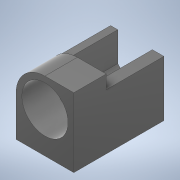
# Autodesk Inventor part: MotorMountV1
Saved by Autodesk Inventor 2020 (Build 240168000, 168)
## iProperties
Created: 2023-11-27
Part Number: MotorMountV1
Material: Thermoplastic Resin
Document SubType Name: Modeling
Designer: smz3rm
Density: 1.28 g/cm^3
Appearance: Smooth - Black
Author: smz3rm
Autodesk Inventor part; units mm, degrees
ref_plane "YZ Plane" through (0, 0, 0) normal (1, 0, 0) x (0, 1, 0)
ref_plane "XZ Plane" through (0, 0, 0) normal (0, 1, 0) x (-1, 0, 0)
ref_plane "XY Plane" through (0, 0, 0) normal (0, 0, 1) x (1, 0, 0)
sketch "Sketch4" plane through (0, 0, 0) normal (0, 0, 1) x (1, 0, 0)
  circle A0 centre (0, 0) radius 8
  circle A1 centre (0, 0) radius 10
  line L0 (-10, 0) -> (-10, -14)
  line L1 (10, 0) -> (10, -14)
  line L2 (10, -14) -> (-10, -14)
  line L3 (10, 0) -> (10, 10)
  line L4 (10, 10) -> (0, 10)
  point P0 (10, -7)
  dimension "d12" = 16
  dimension "d13" = 2
  dimension "d14" = 14
  dimension "d17" = 20
  constraints: 10 end point, 3 point on circle, 2 centre point, 2 vertical, 1 coincident, 1 horizontal, 1 midpoint, 1 perpendicular, 1 point on line, 1 tangent
  measures "d12" diameter of A0
  measures "d13" radial gap between concentric circles of A0 A1
  measures "d14" distance of L0.start L0.end
  measures "d17" distance of L1.end L0.end
extrude "Extrusion3" add sketch "Sketch4" along normal blind 11.25
sketch "Sketch5" plane through (0, 0, 0) normal (0, 0, -1) x (-1, 0, 0)
  circle A0 centre (0, 0) radius 8 projected
  line L0 (0, -19.2142) -> (0, 17.2853) projected
  arc A1 (10, 0) -> (0, 10) centre (0, 0) ccw projected
  line L1 (10, 0) -> (10, -14) projected
  arc A2 (10, 0) -> (0, 10) centre (0, 0) ccw projected
  line L2 (10, -14) -> (-10, -14) projected
  circle A3 centre (0, 0) radius 8 projected
  line L3 (-10, 10) -> (0, 10) projected
  line L4 (-10, -14) -> (-10, 10) projected
  circle A4 centre (0, 0) radius 7.75
  line L5 (-6, -4.9054) -> (-6, 4.9054)
  line L6 (6, -4.9054) -> (6, 4.9054)
  line L7 (-6, 4.9054) -> (-6, 5.2915)
  line L8 (6, 4.9054) -> (6, 5.2915)
  line L9 (-6, 5.2915) -> (-10, 5.2915)
  line L10 (-10, -14) -> (-10, 10) projected
  line L11 (6, 5.2915) -> (8.4853, 5.2915)
  point P0 (-10, 0)
  point P1 (-10, 0)
  dimension "d24" = 15.5
  dimension "d25" = 12
  constraints: 12 end point, 5 point on circle, 3 vertical, 2 point on line, 2 symmetric about line, 1 centre point, 1 coincident, 1 perpendicular
  measures "d24" diameter of A4
  measures "d25" distance between parallel lines of L6 L5
extrude "Extrusion4" add sketch "Sketch5" along normal blind 20 contours A0 L0 A4 L8 | A0 L11 A1 L1 L2 L0 | L0 L2 L4 L9 A0 | A0 L7 A4 L0 | A4 L6 | L5 A4 picked at (6.6814, 4.0106) picked at (-6.667, 4.0378)
equation "\"d14\" = DriveMotorHeight - BaseWallThickness"
equation "\"DriveMotorHeight\" = 17"
equation "\"BaseWallThickness\" = 3"
body "Solid2"
